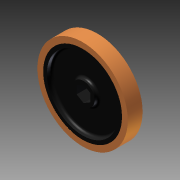
# Autodesk Inventor part: T80P-494BO-HS6
Saved by Autodesk Inventor 2012 (Build 160160000, 160)
## iProperties
Created: 2013-07-13
Part Number: T80P-494BO-HS6
Material: PC_ABS Plastic
Document SubType Name: Modeling
Designer: joe_000
Density: 1.493 g/cm^3
Mass: 228.252 g
Surface Area: 500.925 cm^2
Volume: 152.881 cm^3
Author: joe_000
Autodesk Inventor part; units mm, degrees
ref_plane "YZ Plane" through (0, 0, 0) normal (1, 0, 0) x (0, 1, 0)
ref_plane "XZ Plane" through (0, 0, 0) normal (0, 1, 0) x (-1, 0, 0)
ref_plane "XY Plane" through (0, 0, 0) normal (0, 0, 1) x (1, 0, 0)
sketch "Sketch1" plane through (0, 0, 0) normal (0, 0, 1) x (1, 0, 0)
  line L0 (9.525, 5.4993) -> (9.525, -5.4993)
  line L1 (9.525, -5.4993) -> (0, -10.9985)
  line L2 (0, -10.9985) -> (-9.525, -5.4993)
  line L3 (-9.525, -5.4993) -> (-9.525, 5.4993)
  line L4 (-9.525, 5.4993) -> (0, 10.9985)
  line L5 (0, 10.9985) -> (9.525, 5.4993)
  circle A0 centre (0, 0) radius 53.975
  dimension "d0" = 19.05
  dimension "d1" = 107.95
  constraints: 12 end point, 2 coincident, 1 centre point, 1 vertical, 13 other
  measures "d0" distance between parallel lines of L5 L2
  measures "d1" diameter of A0
extrude "Extrusion1" add sketch "Sketch1" along normal mid plane 7.62
sketch "Sketch3" plane through (0, 0, -3.81) normal (0, 0, -1) x (-1, 0, 0)
  circle A0 centre (0, 0) radius 53.975 projected
  circle A1 centre (0, 0) radius 48.895
  dimension "d7" = 5.08
  constraints: 1 centre point, 1 coincident
  measures "d7" radial gap between concentric circles of A0 A1
extrude "Extrusion3" add sketch "Sketch3" along normal blind 6.35
sketch "Sketch4" plane through (0, 0, 3.81) normal (0, 0, 1) x (1, 0, 0)
  circle A0 centre (0, 0) radius 53.975 projected
  circle A1 centre (0, 0) radius 48.895
  dimension "d10" = 5.08
  constraints: 1 centre point, 1 coincident
  measures "d10" radial gap between concentric circles of A0 A1
extrude "Extrusion4" add sketch "Sketch4" along normal blind 6.35
fillet "Fillet1" radius 3.175 1 edges at (-48.895, 0, 3.81)
fillet "Fillet2" radius 3.175 1 edges at (48.895, 0, -3.81)
sketch "Sketch5" plane through (0, 0, -3.81) normal (0, 0, -1) x (-1, 0, 0)
  line L0 (0, -10.9985) -> (-9.525, -5.4993) projected
  line L1 (-9.525, -5.4993) -> (-9.525, 5.4993) projected
  line L2 (-9.525, 5.4993) -> (0, 10.9985) projected
  line L3 (0, 10.9985) -> (9.525, 5.4993) projected
  line L4 (9.525, 5.4993) -> (9.525, -5.4993) projected
  line L5 (9.525, -5.4993) -> (0, -10.9985) projected
  circle A0 centre (0, 0) radius 45.72 projected
  circle A1 centre (0, 0) radius 15.24
  dimension "d15" = 30.48
  constraints: 1 centre point, 1 coincident
  measures "d15" diameter of A1
extrude "Extrusion5" add sketch "Sketch5" along normal blind 5.08 contours A1
fillet "Fillet3" radius 3.175 1 edges at (15.24, 0, -3.81)
sketch "Sketch6" plane through (0, 0, 3.81) normal (0, 0, 1) x (1, 0, 0)
  line L0 (9.525, -5.4993) -> (0, -10.9985) projected
  line L1 (0, -10.9985) -> (-9.525, -5.4993) projected
  line L2 (-9.525, -5.4993) -> (-9.525, 5.4993) projected
  line L3 (-9.525, 5.4993) -> (0, 10.9985) projected
  line L4 (0, 10.9985) -> (9.525, 5.4993) projected
  line L5 (9.525, 5.4993) -> (9.525, -5.4993) projected
  circle A0 centre (0, 0) radius 45.72 projected
  circle A1 centre (0, 0) radius 15.24
  dimension "d19" = 30.48
  constraints: 1 centre point, 1 coincident
  measures "d19" diameter of A1
extrude "Extrusion6" add sketch "Sketch6" along normal blind 5.08 contours A1
fillet "Fillet4" radius 3.175 1 edges at (-15.24, 0, 3.81)
sketch "Sketch7" plane through (0, 0, 0) normal (0, 0, 1) x (1, 0, 0)
  circle A0 centre (0, 0) radius 61.9125
  circle A1 centre (0, 0) radius 53.975
  circle A2 centre (0, 0) radius 53.975 projected
  dimension "d23" = 123.825
  constraints: 2 centre point, 2 coincident, 1 concentric
  measures "d23" diameter of A0
extrude "Extrusion7" add sketch "Sketch7" along normal mid plane 20.32 separate body
body "Solid2"
